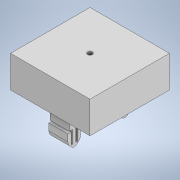
# Autodesk Inventor part: SiPM outer housing
Saved by Autodesk Inventor 2020 (Build 240168000, 168)
## iProperties
Created: 2021-06-25
Part Number: SiPM outer housing
Material: Generic
Document SubType Name: Modeling
Designer: alejandrosalazar
Density: 1 g/cm^3
Appearance: Default
Author: alejandrosalazar
Autodesk Inventor part; units mm, degrees
ref_plane "YZ Plane" through (0, 0, 0) normal (1, 0, 0) x (0, 1, 0)
ref_plane "XZ Plane" through (0, 0, 0) normal (0, 1, 0) x (-1, 0, 0)
ref_plane "XY Plane" through (0, 0, 0) normal (0, 0, 1) x (1, 0, 0)
sketch "Sketch1" plane through (0, 0, 0) normal (0, 1, 0) x (-1, 0, 0)
  line L0 (0, 0) -> (-25, 0)
  line L1 (-25, 0) -> (-25, 25)
  line L2 (-25, 25) -> (0, 25)
  line L3 (0, 25) -> (0, 0)
  circle A0 centre (-4.5, 4.5) radius 4
  circle A1 centre (-4.5, 20.5) radius 4
  circle A2 centre (-20.5, 20.5) radius 4
  circle A3 centre (-20.5, 4.5) radius 4
  dimension "d0" = 25
  dimension "d1" = 25
  dimension "d2" = 8
  dimension "d3" = 8
  dimension "d4" = 8
  dimension "d5" = 8
  constraints: 8 end point, 4 centre point, 2 parallel, 1 horizontal, 1 perpendicular
  measures "d0" distance of L1.end L2.end
  measures "d1" distance of L0.end L1.end
  measures "d2" diameter of A0
  measures "d3" diameter of A1
  measures "d4" diameter of A2
  measures "d5" diameter of A3
extrude "Extrusion1" add sketch "Sketch1" along normal blind 5
sketch "Sketch2" plane through (0, 5, 0) normal (0, 1, 0) x (1, 0, 0)
  line L0 (0, 0) -> (0, -25) projected
  line L1 (25, -25) -> (25, 0) projected
  line L2 (0, -25) -> (25, -25)
  line L3 (25, -25) -> (25, 0)
  line L4 (25, 0) -> (0, 0)
  line L5 (0, 0) -> (0, -25)
  constraints: 8 end point, 2 parallel, 1 horizontal, 1 perpendicular
extrude "Extrusion2" add sketch "Sketch2" along normal blind 5
sketch "Sketch4" plane through (0, 0, 0) normal (0, -1, 0) x (1, 0, 0)
  line L0 (9.5, 3) -> (15.5, 3)
  line L1 (15.5, 3) -> (15.5, 6)
  line L2 (15.5, 6) -> (9.5, 6)
  line L3 (9.5, 6) -> (9.5, 3)
  line L4 (9.5, 22) -> (15.5, 22)
  line L5 (15.5, 22) -> (15.5, 19)
  line L6 (15.5, 19) -> (9.5, 19)
  line L7 (9.5, 19) -> (9.5, 22)
  point P0 (0, 0)
  dimension "d12" = 6
  dimension "d13" = 3
  dimension "d14" = 6
  dimension "d15" = 3
  constraints: 16 end point, 4 parallel, 2 horizontal, 2 perpendicular, 1 point on line
  measures "d12" distance of L2.end L1.end
  measures "d13" distance of L1.end L0.end
  measures "d14" distance of L5.end L6.end
  measures "d15" distance of L4.end L5.end
extrude "Extrusion3" add sketch "Sketch4" along normal blind 5
sketch "Sketch5" plane through (0, -5, 0) normal (0, -1, 0) x (1, 0, 0)
  line L0 (15.5, 3) -> (15.5, 6) projected
  line L1 (9.5, 6) -> (9.5, 3) projected
  line L2 (15.5, 4) -> (9.5, 4)
  line L3 (9.5, 4) -> (9.5, 5)
  line L4 (9.5, 5) -> (15.5, 5)
  line L5 (15.5, 5) -> (15.5, 4)
  line L6 (15.5, 19) -> (15.5, 22) projected
  line L7 (15.5, 21) -> (9.5, 21)
  line L8 (9.5, 21) -> (9.5, 20)
  line L9 (9.5, 20) -> (15.5, 20)
  line L10 (15.5, 20) -> (15.5, 21)
  point P0 (0, 0)
  dimension "d18" = 1
  dimension "d19" = 6
  dimension "d20" = 1
  constraints: 16 end point, 4 parallel, 3 point on line, 2 horizontal, 2 perpendicular
  measures "d18" distance of L2.end L3.end
  measures "d19" distance of L9.end L8.end
  measures "d20" distance of L8.end L7.end
extrude "Extrusion4" add sketch "Sketch5" along normal blind 4
sketch "Sketch6" plane through (0, -9, 0) normal (0, -1, 0) x (1, 0, 0)
  line L0 (15.5, 6) -> (15.5, 3) projected
  line L1 (9.5, 3) -> (9.5, 6) projected
  line L2 (15.5, 5.5) -> (9.5, 5.5)
  line L3 (9.5, 5.5) -> (9.5, 3.5)
  line L4 (9.5, 3.5) -> (15.5, 3.5)
  line L5 (15.5, 3.5) -> (15.5, 5.5)
  line L6 (15.5, 22) -> (15.5, 19) projected
  line L7 (15.5, 21.45) -> (9.5, 21.45)
  line L8 (9.5, 21.45) -> (9.5, 19.45)
  line L9 (9.5, 19.45) -> (15.5, 19.45)
  line L10 (15.5, 19.45) -> (15.5, 21.45)
  point P0 (0, 0)
  dimension "d23" = 2
  dimension "d24" = 6
  dimension "d25" = 2
  constraints: 16 end point, 4 parallel, 3 point on line, 2 horizontal, 2 perpendicular
  measures "d23" distance of L3.end L2.end
  measures "d24" distance of L9.end L8.end
  measures "d25" distance of L8.end L7.end
extrude "Extrusion5" add sketch "Sketch6" along normal blind 1
sketch "Sketch7" plane through (15.5, -9, 19.45) normal (0, 0, -1) x (-1, 0, 0)
  line L0 (0, 0) -> (0, -1) projected
  line L1 (6, 4) -> (6, 0) projected
  line L2 (0, -1) -> (6, -1)
  line L3 (6, -1) -> (6, 3.5)
  line L4 (6, 3.5) -> (0, 3.5)
  line L5 (0, 3.5) -> (0, -1)
  point P0 (15.5, 9)
  dimension "d28" = 4.5
  constraints: 8 end point, 2 parallel, 1 horizontal, 1 perpendicular, 1 point on line
  measures "d28" distance of L3.end L2.end
extrude "Extrusion6" add sketch "Sketch7" along normal blind 1
sketch "Sketch8" plane through (9.5, -9, 21.45) normal (0, 0, 1) x (1, 0, 0)
  line L0 (6, 0) -> (6, -1) projected
  line L1 (0, 4) -> (0, 0) projected
  line L2 (6, -1) -> (0, -1)
  line L3 (0, -1) -> (0, 3.5)
  line L4 (0, 3.5) -> (6, 3.5)
  line L5 (6, 3.5) -> (6, -1)
  point P0 (-9.5, 9)
  dimension "d31" = 4.5
  constraints: 8 end point, 2 parallel, 1 horizontal, 1 perpendicular, 1 point on line
  measures "d31" distance of L2.end L3.end
extrude "Extrusion7" add sketch "Sketch8" along normal blind 1
sketch "Sketch9" plane through (9.5, -9, 5.5) normal (0, 0, 1) x (1, 0, 0)
  line L0 (6, -1) -> (0, -1) projected
  line L1 (0, 4) -> (0, 0) projected
  line L2 (6, -1) -> (0, -1)
  line L3 (0, -1) -> (0, 3.5)
  line L4 (0, 3.5) -> (6, 3.5)
  line L5 (6, 3.5) -> (6, -1)
  point P0 (-9.5, 9)
  dimension "d34" = 4.5
  constraints: 8 end point, 2 parallel, 1 horizontal, 1 perpendicular, 1 point on line
  measures "d34" distance of L2.end L3.end
extrude "Extrusion8" add sketch "Sketch9" along normal blind 1
sketch "Sketch10" plane through (15.5, -9, 3.5) normal (0, 0, -1) x (-1, 0, 0)
  line L0 (6, 0) -> (6, -1) projected
  line L1 (0, 3.5) -> (6, 3.5) projected
  line L2 (6, -1) -> (0, -1)
  line L3 (0, -1) -> (0, 3.5)
  line L4 (0, 3.5) -> (6, 3.5)
  line L5 (6, 3.5) -> (6, -1)
  point P0 (15.5, 9)
  dimension "d37" = 4.5
  constraints: 8 end point, 2 parallel, 1 horizontal, 1 perpendicular
  measures "d37" distance of L2.end L1.start
extrude "Extrusion9" add sketch "Sketch10" along normal blind 1
chamfer "Chamfer1" distance 1.5 angle 45 1 edges at (12.5, -10, 2.5)
chamfer "Chamfer2" distance 1.5 angle 45 1 edges at (12.5, -10, 6.5)
fillet "Fillet1" radius 2 2 edges at (12.5, -8.5, 2.5) (12.5, -8.5, 6.5)
fillet "Fillet2" radius 1 2 edges at (12.5, -10, 5) (12.5, -10, 4)
chamfer "Chamfer3" distance 1.5 angle 45 2 edges at (12.5, -10, 18.45) (12.5, -10, 22.45)
fillet "Fillet3" radius 1 2 edges at (12.5, -10, 20.95) (12.5, -10, 19.95)
fillet "Fillet4" radius 2 2 edges at (12.5, -8.5, 22.45) (12.5, -8.5, 18.45)
sketch "Sketch11" plane through (0, 10, 0) normal (0, 1, 0) x (1, 0, 0)
  circle A0 centre (12.5, -12.5) radius 0.75
  point P0 (0, 0)
  dimension "d53" = 1.5
  constraints: 1 centre point
  measures "d53" diameter of A0
hole "Hole1" at (12.5, 10, 12.5) direction (0, -1, 0) diameter 1.5 depth 10
body "Solid1"
